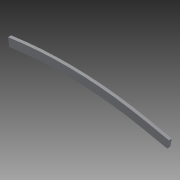
# Autodesk Inventor part: nd-i
Saved by Autodesk Inventor 2015 (Build 190159000, 159)
## iProperties
Created: 2014-07-02
Part Number: nd-i
Material: Generic
Document SubType Name: Modeling
Designer: peter
Density: 1 g/cm^3
Appearance: Default
Author: peter
Autodesk Inventor part; units mm, degrees
ref_plane "YZ Plane" through (0, 0, 0) normal (1, 0, 0) x (0, 1, 0)
ref_plane "XZ Plane" through (0, 0, 0) normal (0, 1, 0) x (-1, 0, 0)
ref_plane "XY Plane" through (0, 0, 0) normal (0, 0, 1) x (1, 0, 0)
sketch "Sketch1" plane through (0, 0, 0) normal (0, 0, 1) x (1, 0, 0)
  line L0 (0.0002, 105.7836) -> (7.461, 55.5344)
  arc A0 (845.4951, 31.1517) -> (7.461, 55.5344) centre (358.1185, -2306.1754) ccw
  line L1 (845.4951, 31.1517) -> (994.6862, 0.0425)
  line L2 (994.6862, 0.0425) -> (1005.0559, 49.7729)
  line L3 (1005.0559, 49.7729) -> (855.8648, 80.8821)
  arc A1 (855.8648, 80.8821) -> (0.0002, 105.7836) centre (358.1185, -2306.1754) ccw
  constraints: 8 end point, 4 point on circle, 2 centre point
extrude "Extrusion1" add sketch "Sketch1" along normal blind 19.05
body "Solid1"
